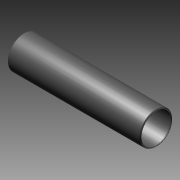
# Autodesk Inventor part: 17R-6.30250C
Saved by Autodesk Inventor 2011 SP1 (Build 150282100, 282)
## iProperties
Created: 2016-10-01
Part Number: 17R-6.30250C
Catalog Web Link: www.cadenas.de
Description: Tube-Original Line - Standard Air Cylinders
Vendor: BIMBA
Document SubType Name: Modeling
Designer: psAdmin
Manufacturer: BIMBA
Mass: 11.5043 g
Surface Area: 398.733 cm^2
Volume: 11.5043 cm^3
Density: 1 g/cm^3
Category: PARTsolutions
Company: BIMBA
Title: 17R-6.30250C
Author: Cadenas PARTsolutions
Comments: Original Line - Standard Air Cylinders
PSOL_IDENT_0: {$CADENAS_DATA\23d-libs\bimba\bimba\bimba_imperial\bimba_full_line\original_line_cylinders\standard_
PSOL_IDENT_1: air_cylinders\tube.prj},192 {VTYP=3D},{NB=17R-6.30250C},{LINA=17R-6.30250C},{NN=Tube},{DATE=22.09.20
PSOL_IDENT_2: 16 13:52:25},{GEOMDATE=18.02.2011 00:00:00},{VERSION=},{LINEID=80},{LINESUBID=-1},{WBVAR=MNT,ACTING,
PSOL_IDENT_3: NR,L,FOURHOLES,SR}  {NB=17R-6.30250C},{LINA=17R-6.30250C},{KT=DUMMY},{PN=17R-6.30250C},{BORE=1.50000
PSOL_IDENT_4: 000},{BOREPN=17},{MNT=},{MNTALG='' , 'Front Nose' , 'BF' , 'Front Block' , 'BFT' , 'Front Trunnion'
PSOL_IDENT_5: , 'A' , 'Adjustable Stroke'},{ACTING=R},{ACTINGALG= '' , 'Single Acting' , 'R' , 'Reverse/Double Act
PSOL_IDENT_6: ing' },{NR=},{NRALG= '' , 'Without Non-rotating Rod' , 'NR' , 'With Non-rotating Rod' },{L=6.3025},{
PSOL_IDENT_7: OD=1.5565},{ODN=1.5565},{ODP=1.5565},{ODB=1.5800},{ID=1.5115},{DV=0.00000000},{LV=0.00000000},{LV1=0
PSOL_IDENT_8: .00000000},{G=0.0400},{FOURHOLES=0},{AA=0.3750},{BB=0.1250},{SR=C},{SRALG= 'C' , 'Carbon Steel Rod'
PSOL_IDENT_9: , 'SR' , '303 Stainless Steel Rod' , '' , '303 Stainless Steel Rod'}
NN: Tube
NT: Original Line - Standard Air Cylinders
NB: 17R-6.30250C
NBSYN: $PN.
LINA: 17R-6.30250C
BORE: 1 1/2
BOREPN: 17
MNT: Front Nose
MNTALG: '' , 'Front Nose' , 'BF' , 'Front Block' , 'BFT' , 'Front Trunnion' , 'A' , 'Adjustable Stroke'
ACTING: Reverse/Double Acting
NR: Without Non-rotating Rod
L: 6.3025
ODN: 1.5565
ODP: 1.5565
ODB: 1.5800
ID: 1.5115
DV: 0.00000000
LV: 0.00000000
LV1: 0.00000000
G: 0.0400
FOURHOLES: 0
AA: 0.3750
BB: 0.1250
SR: Carbon Steel Rod
SUPPLIER: BIMBA
ARTICLENO: 17R-6.30250C
BOMINFO: 17R-6.30250C
CREATOR: CADENAS GmbH
Autodesk Inventor part; units mm, degrees
ref_plane "YZ Plane" through (0, 0, 0) normal (1, 0, 0) x (0, 1, 0)
ref_plane "XZ Plane" through (0, 0, 0) normal (0, 1, 0) x (-1, 0, 0)
ref_plane "XY Plane" through (0, 0, 0) normal (0, 0, 1) x (1, 0, 0)
sketch "Sketch_1" plane through (0, 0, 0) normal (0, 0, 1) x (1, 0, 0)
  line L0 (160.0835, 0) -> (0, 0)
  arc A0 (-0.8826, 18.7343) -> (-0.8826, 18.5547) centre (-0.7928, 18.6445) ccw
  line L1 (-0.8826, 18.5547) -> (-0.508, 18.1801)
  line L2 (-0.508, 18.1801) -> (0, 18.1801)
  line L3 (0, 18.1801) -> (1.016, 19.196)
  line L4 (1.016, 19.196) -> (159.0675, 19.196)
  line L5 (159.0675, 19.196) -> (160.0835, 18.1801)
  line L6 (160.0835, 18.1801) -> (160.5915, 18.1801)
  line L7 (160.5915, 18.1801) -> (160.9661, 18.5547)
  arc A1 (160.9661, 18.5547) -> (160.9661, 18.7343) centre (160.8763, 18.6445) ccw
  line L8 (160.9661, 18.7343) -> (160.2304, 19.47)
  arc A2 (160.2304, 19.47) -> (159.512, 19.7675) centre (159.512, 18.7515) ccw
  line L9 (159.512, 19.7675) -> (0.5715, 19.7675)
  arc A3 (0.5715, 19.7675) -> (-0.1469, 19.47) centre (0.5715, 18.7515) ccw
  line L10 (-0.1469, 19.47) -> (-0.8826, 18.7343)
  constraints: 22 end point, 8 point on circle, 4 centre point
revolve "Revolution1" add sketch "Sketch_1" angle 360 about axis through (160.0835, 0, 0) along (1, 0, 0)
ref_plane "cp1_XY" through (80.0418, 19.7675, 0) normal (1, 0, 0) x (0, 0, -1)
ref_plane "cp1_YZ" through (80.0418, 19.7675, 0) normal (0, 0, -1) x (0, 1, 0)
ref_plane "cp1_ZX" through (80.0418, 19.7675, 0) normal (0, 1, 0) x (1, 0, 0)
ref_plane "cp2_XY" through (80.0418, 0, -19.7675) normal (1, 0, 0) x (0, 0, -1)
ref_plane "cp2_YZ" through (80.0418, 0, -19.7675) normal (0, 0, -1) x (0, 1, 0)
ref_plane "cp2_ZX" through (80.0418, 0, -19.7675) normal (0, 1, 0) x (1, 0, 0)
ref_plane "cp3_XY" through (80.0418, -19.7675, 0) normal (1, 0, 0) x (0, 0, -1)
ref_plane "cp3_YZ" through (80.0418, -19.7675, 0) normal (0, 0, -1) x (0, 1, 0)
ref_plane "cp3_ZX" through (80.0418, -19.7675, 0) normal (0, 1, 0) x (1, 0, 0)
ref_plane "cp4_XY" through (80.0418, 0, 19.7675) normal (1, 0, 0) x (0, 0, -1)
ref_plane "cp4_YZ" through (80.0418, 0, 19.7675) normal (0, 0, -1) x (0, 1, 0)
ref_plane "cp4_ZX" through (80.0418, 0, 19.7675) normal (0, 1, 0) x (1, 0, 0)
ref_plane "tube_front_XY" through (0, 0, 0) normal (1, 0, 0) x (0, 0, -1)
ref_plane "tube_front_YZ" through (0, 0, 0) normal (0, 0, -1) x (0, 1, 0)
ref_plane "tube_front_ZX" through (0, 0, 0) normal (0, 1, 0) x (1, 0, 0)
ref_plane "tube_rear_XY" through (160.0835, 0, 0) normal (1, 0, 0) x (0, 0, -1)
ref_plane "tube_rear_YZ" through (160.0835, 0, 0) normal (0, 0, -1) x (0, 1, 0)
ref_plane "tube_rear_ZX" through (160.0835, 0, 0) normal (0, 1, 0) x (1, 0, 0)
body "Solid1"
